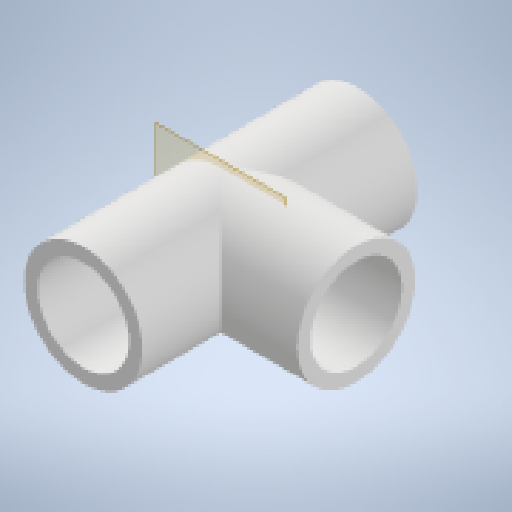
# Autodesk Inventor part: T_PVC
Saved by Autodesk Inventor 2023.1 (Build 271208000, 208)
## iProperties
Created: 2022-08-28
Part Number: T_PVC
Material: Generic
Document SubType Name: Modeling
Designer: Daniel Peña
Density: 1 g/cm^3
Appearance: Default
Author: Daniel Peña
Autodesk Inventor part; units mm, degrees
ref_plane "YZ Plane" through (0, 0, 0) normal (1, 0, 0) x (0, 1, 0)
ref_plane "XZ Plane" through (0, 0, 0) normal (0, 1, 0) x (-1, 0, 0)
ref_plane "XY Plane" through (0, 0, 0) normal (0, 0, 1) x (1, 0, 0)
sketch "Sketch1" plane through (0, 0, 0) normal (0, 1, 0) x (-1, 0, 0)
  line L0 (12.4164, 29.1571) -> (12.4164, -28.0429)
  line L1 (26.4164, 20.9161) -> (23.2164, 20.9161)
  line L2 (23.2164, -44.0839) -> (26.4164, -44.0839)
  line L3 (26.4164, -44.0839) -> (26.4164, 20.9161)
  line L4 (23.2164, -24.0839) -> (22.8164, -24.0839)
  line L5 (22.8164, -24.0839) -> (22.8164, -23.5843)
  line L6 (22.8164, -23.5843) -> (23.2164, -23.5843)
  line L7 (23.2164, 0.9161) -> (22.8164, 0.9161)
  line L8 (22.8164, 0.9161) -> (22.8164, 0.4161)
  line L9 (22.8164, 0.4161) -> (23.2164, 0.4161)
  line L10 (23.2164, 20.9161) -> (23.2164, 0.9161)
  line L11 (23.2164, 0.4161) -> (23.2164, -23.5843)
  line L12 (23.2164, -24.0839) -> (23.2164, -44.0839)
  point P0 (0, 0)
  dimension "d0" = 65
  dimension "d1" = 3.2
  dimension "d3" = 20
  dimension "d4" = 0.4
  dimension "d6" = 20
  dimension "d7" = 28
  dimension "d8" = 0.5
  dimension "d9" = 0.4
  constraints: 26 end point, 5 parallel, 5 perpendicular, 3 horizontal, 2 vertical
  measures "d0" distance of L2.end L1.start
  measures "d1" distance of L2.start L2.end
  measures "d3" distance between parallel lines of L2 L4
  measures "d4" distance of L9.end L8.end
  measures "d6" distance between parallel lines of L1 L7
  measures "d7" diameter of L3 L0
  measures "d8" distance of L7.end L8.end
  measures "d9" distance between parallel lines of L12 L5
revolve "Revolution1" add sketch "Sketch1" angle 360 about axis through (-12.4164, 0, 29.1571) along (0, 0, -1)
ref_plane "Work Plane1" through (-12.4164, 0, -11.5839) normal (0, 0, 1) x (1, 0, 0)
sketch "Sketch2" plane through (-12.4164, 0, -11.5839) normal (0, 0, 1) x (1, 0, 0)
  line L0 (10.4389, 0) -> (54.145, 0)
  circle A0 centre (0, 0) radius 14 projected
  line L1 (0, 10.8) -> (0, 14)
  line L2 (0, 14) -> (32, 14)
  line L3 (32, 14) -> (32, 10.8)
  line L4 (11.5, 10.8) -> (11.5, 10.4)
  line L5 (11.5, 10.4) -> (12, 10.4)
  line L6 (12, 10.4) -> (12, 10.8)
  line L7 (32, 10.8) -> (12, 10.8)
  line L8 (11.5, 10.8) -> (0, 10.8)
  line L9 (-14, 0) -> (-14, 10.4)
  point P0 (12.4164, 0)
  point P1 (8.9084, 10.8)
  dimension "d11" = 28
  dimension "d12" = 3.2
  dimension "d13" = 0.5
  dimension "d14" = 0.4
  dimension "d15" = 20
  dimension "d16" = 46
  constraints: 20 end point, 4 parallel, 3 horizontal, 2 perpendicular, 2 point on circle, 1 tangent, 1 vertical
  measures "d11" diameter of L2 L0
  measures "d12" distance of L2.end L3.end
  measures "d13" distance of L5.end L4.end
  measures "d14" distance of L4.end L4.start
  measures "d15" distance between parallel lines of L3 L6
  measures "d16" distance between parallel lines of L3 L9
revolve "Revolution2" add sketch "Sketch2" angle 360 about axis through (-1.9774, 0, -11.5839) along (1, 0, 0) contours L2 L3 L7 L6 L5 L4 L8 A0
sketch "Sketch4" plane through (-12.4164, 0, -44.0839) normal (0, 0, -1) x (-1, 0, 0)
  circle A0 centre (0, 0) radius 10.4
  point P0 (-12.4164, 0)
  constraints: 1 centre point
extrude "Extrusion1" cut sketch "Sketch4" against normal up to surface (65 mm away)
sketch "Sketch5" plane through (19.5836, 0, -11.5839) normal (1, 0, 0) x (0, 0, -1)
  arc A0 (-7.494, -7.2111) -> (7.494, -7.2111) centre (0, 0) ccw projected
  circle A1 centre (0, 0) radius 10.4
  point P0 (-11.5839, 0)
  point P1 (7.494, -7.2111)
  constraints: 3 other
extrude "Extrusion2" cut sketch "Sketch5" against normal up to surface
body "Solid1"
